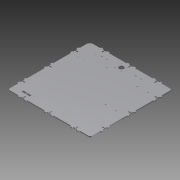
# Autodesk Inventor part: base
Saved by Autodesk Inventor 2012 (Build 160160000, 160)
## iProperties
Created: 2014-12-15
Part Number: base
Material: Default
Document SubType Name: Modeling
Designer: PRINCIPAL
Density: 1 g/cm^3
Author: PRINCIPAL
Autodesk Inventor part; units mm, degrees
ref_plane "YZ Plane" through (0, 0, 0) normal (1, 0, 0) x (0, 1, 0)
ref_plane "XZ Plane" through (0, 0, 0) normal (0, 1, 0) x (-1, 0, 0)
ref_plane "XY Plane" through (0, 0, 0) normal (0, 0, 1) x (1, 0, 0)
sketch "Boceto1" plane through (0, 0, 0) normal (0, 0, 1) x (1, 0, 0)
  arc A0 (118.25, 311.375) -> (118.25, 314.525) centre (118.25, 312.95) ccw
  line L0 (118.25, 311.375) -> (114.65, 311.375)
  arc A1 (114.65, 314.525) -> (114.65, 311.375) centre (114.65, 312.95) ccw
  line L1 (114.65, 314.525) -> (118.25, 314.525)
  arc A2 (93.2214, 311.4) -> (93.2214, 314.5) centre (93.2214, 312.95) ccw
  line L2 (93.2214, 311.4) -> (89.6786, 311.4)
  arc A3 (89.6786, 314.5) -> (89.6786, 311.4) centre (89.6786, 312.95) ccw
  line L3 (89.6786, 314.5) -> (93.2214, 314.5)
  line L4 (251.6786, 314.5) -> (255.2214, 314.5)
  arc A4 (255.2214, 311.4) -> (255.2214, 314.5) centre (255.2214, 312.95) ccw
  line L5 (255.2214, 311.4) -> (251.6786, 311.4)
  arc A5 (251.6786, 314.5) -> (251.6786, 311.4) centre (251.6786, 312.95) ccw
  line L6 (276.6786, 314.5) -> (280.2214, 314.5)
  arc A6 (280.2214, 311.4) -> (280.2214, 314.5) centre (280.2214, 312.95) ccw
  line L7 (280.2214, 311.4) -> (276.6786, 311.4)
  arc A7 (276.6786, 314.5) -> (276.6786, 311.4) centre (276.6786, 312.95) ccw
  arc A8 (184.95, 323.95) -> (173.95, 312.95) centre (184.95, 312.95) ccw
  arc A9 (173.95, 312.95) -> (184.95, 301.95) centre (184.95, 312.95) ccw
  arc A10 (184.95, 301.95) -> (195.95, 312.95) centre (184.95, 312.95) ccw
  arc A11 (195.95, 312.95) -> (184.95, 323.95) centre (184.95, 312.95) ccw
  arc A12 (169.45, 299) -> (167.9, 297.45) centre (169.45, 297.45) ccw
  arc A13 (167.9, 297.45) -> (169.45, 295.9) centre (169.45, 297.45) ccw
  arc A14 (169.45, 295.9) -> (171, 297.45) centre (169.45, 297.45) ccw
  arc A15 (171, 297.45) -> (169.45, 299) centre (169.45, 297.45) ccw
  arc A16 (200.45, 330) -> (198.9, 328.45) centre (200.45, 328.45) ccw
  arc A17 (198.9, 328.45) -> (200.45, 326.9) centre (200.45, 328.45) ccw
  arc A18 (200.45, 326.9) -> (202, 328.45) centre (200.45, 328.45) ccw
  arc A19 (202, 328.45) -> (200.45, 330) centre (200.45, 328.45) ccw
  arc A20 (169.45, 330) -> (167.9, 328.45) centre (169.45, 328.45) ccw
  arc A21 (167.9, 328.45) -> (169.45, 326.9) centre (169.45, 328.45) ccw
  arc A22 (169.45, 326.9) -> (171, 328.45) centre (169.45, 328.45) ccw
  arc A23 (171, 328.45) -> (169.45, 330) centre (169.45, 328.45) ccw
  arc A24 (200.45, 299) -> (198.9, 297.45) centre (200.45, 297.45) ccw
  arc A25 (198.9, 297.45) -> (200.45, 295.9) centre (200.45, 297.45) ccw
  arc A26 (200.45, 295.9) -> (202, 297.45) centre (200.45, 297.45) ccw
  arc A27 (202, 297.45) -> (200.45, 299) centre (200.45, 297.45) ccw
  line L8 (197.9907, 331.1677) -> (197.9907, 334.0126)
  line L9 (197.9907, 334.0126) -> (196.7407, 334.0126)
  line L10 (196.7407, 334.0126) -> (196.7407, 337)
  line L11 (196.7407, 337) -> (197.9907, 337)
  line L12 (197.9907, 337) -> (197.9907, 342.9)
  line L13 (197.9907, 342.9) -> (190.1, 342.9)
  line L14 (190.1, 342.9) -> (190.1, 347.9)
  line L15 (190.1, 347.9) -> (179.8, 347.9)
  line L16 (179.8, 347.9) -> (179.8, 342.9)
  line L17 (179.8, 342.9) -> (95.1, 342.9)
  line L18 (95.1, 342.9) -> (95.1, 347.9)
  line L19 (95.1, 347.9) -> (84.8, 347.9)
  line L20 (84.8, 347.9) -> (84.8, 342.9)
  line L21 (84.8, 342.9) -> (77.1372, 342.9)
  line L22 (77.1372, 342.9) -> (77.1372, 337)
  line L23 (77.1372, 337) -> (78.3872, 337)
  line L24 (78.3872, 337) -> (78.3872, 334.0126)
  line L25 (78.3872, 334.0126) -> (77.1372, 334.0126)
  line L26 (77.1372, 334.0126) -> (77.1372, 329.7126)
  line L27 (77.1372, 329.7126) -> (72.9907, 329.7126)
  line L28 (72.9907, 329.7126) -> (72.9907, 334.0126)
  line L29 (72.9907, 334.0126) -> (71.7407, 334.0126)
  line L30 (71.7407, 334.0126) -> (71.7407, 337)
  line L31 (71.7407, 337) -> (72.9907, 337)
  line L32 (72.9907, 337) -> (72.9907, 342.9)
  line L33 (72.9907, 342.9) -> (65.1, 342.9)
  line L34 (65.1, 342.9) -> (65.1, 347.9)
  line L35 (65.1, 347.9) -> (54.8, 347.9)
  line L36 (54.8, 347.9) -> (54.8, 342.9)
  line L37 (54.8, 342.9) -> (20, 342.9)
  arc A28 (20, 342.9) -> (5, 327.9) centre (20, 327.9) ccw
  line L38 (5, 327.9) -> (5, 294.1)
  line L39 (5, 294.1) -> (0, 294.1)
  line L40 (0, 294.1) -> (0, 283.8)
  line L41 (0, 283.8) -> (5, 283.8)
  line L42 (5, 283.8) -> (5, 275.9744)
  line L43 (5, 275.9744) -> (11.0499, 275.9744)
  line L44 (11.0499, 275.9744) -> (11.0499, 277.2244)
  line L45 (11.0499, 277.2244) -> (14.0508, 277.2244)
  line L46 (14.0508, 277.2244) -> (14.0508, 275.9744)
  line L47 (14.0508, 275.9744) -> (18.5, 275.9744)
  line L48 (18.5, 275.9744) -> (18.5, 271.8605)
  line L49 (18.5, 271.8605) -> (14.0508, 271.8605)
  line L50 (14.0508, 271.8605) -> (14.0508, 270.6105)
  line L51 (14.0508, 270.6105) -> (11.0499, 270.6105)
  line L52 (11.0499, 270.6105) -> (11.0499, 271.8605)
  line L53 (11.0499, 271.8605) -> (5, 271.8605)
  line L54 (5, 271.8605) -> (5, 264.1)
  line L55 (5, 264.1) -> (0, 264.1)
  line L56 (0, 264.1) -> (0, 253.8)
  line L57 (0, 253.8) -> (5, 253.8)
  line L58 (5, 253.8) -> (5, 169.1)
  line L59 (5, 169.1) -> (0, 169.1)
  line L60 (0, 169.1) -> (0, 158.8)
  line L61 (0, 158.8) -> (5, 158.8)
  line L62 (5, 158.8) -> (5, 150.9744)
  line L63 (5, 150.9744) -> (11.0501, 150.9744)
  line L64 (11.0501, 150.9744) -> (11.0501, 152.2244)
  line L65 (11.0501, 152.2244) -> (14.0502, 152.2244)
  line L66 (14.0502, 152.2244) -> (14.0502, 150.9744)
  line L67 (14.0502, 150.9744) -> (18.5, 150.9744)
  line L68 (18.5, 150.9744) -> (18.5, 146.8605)
  line L69 (18.5, 146.8605) -> (14.0502, 146.8605)
  line L70 (14.0502, 146.8605) -> (14.0502, 145.6105)
  line L71 (14.0502, 145.6105) -> (11.0501, 145.6105)
  line L72 (11.0501, 145.6105) -> (11.0501, 146.8605)
  line L73 (11.0501, 146.8605) -> (5, 146.8605)
  line L74 (5, 146.8605) -> (5, 139.1)
  line L75 (5, 139.1) -> (0, 139.1)
  line L76 (0, 139.1) -> (0, 128.8)
  line L77 (0, 128.8) -> (5, 128.8)
  line L78 (5, 128.8) -> (5, 44.074)
  line L79 (5, 44.074) -> (0, 44.074)
  line L80 (0, 44.074) -> (0, 33.774)
  line L81 (0, 33.774) -> (5, 33.774)
  line L82 (5, 33.774) -> (5, 25.9484)
  line L83 (5, 25.9484) -> (11.0521, 25.9484)
  line L84 (11.0521, 25.9484) -> (11.0521, 27.1984)
  line L85 (11.0521, 27.1984) -> (14.0499, 27.1984)
  line L86 (14.0499, 27.1984) -> (14.0499, 25.9484)
  line L87 (14.0499, 25.9484) -> (18.3499, 25.9484)
  line L88 (18.3499, 25.9484) -> (18.3499, 21.8345)
  line L89 (18.3499, 21.8345) -> (14.0499, 21.8345)
  line L90 (14.0499, 21.8345) -> (14.0499, 20.5845)
  line L91 (14.0499, 20.5845) -> (11.0521, 20.5845)
  line L92 (11.0521, 20.5845) -> (11.0521, 21.8345)
  line L93 (11.0521, 21.8345) -> (5, 21.8345)
  line L94 (5, 21.8345) -> (5, 14.074)
  line L95 (5, 14.074) -> (0, 14.074)
  line L96 (0, 14.074) -> (0, 3.774)
  line L97 (0, 3.774) -> (5, 3.774)
  line L98 (5, 3.774) -> (5, -37.026)
  arc A29 (5, -37.026) -> (13, -45.026) centre (13, -37.026) ccw
  line L99 (13, -45.026) -> (54.8, -45.026)
  line L100 (54.8, -45.026) -> (54.8, -50.026)
  line L101 (54.8, -50.026) -> (65.1, -50.026)
  line L102 (65.1, -50.026) -> (65.1, -45.026)
  line L103 (65.1, -45.026) -> (72.9907, -45.026)
  line L104 (72.9907, -45.026) -> (72.9907, -39.126)
  line L105 (72.9907, -39.126) -> (71.7407, -39.126)
  line L106 (71.7407, -39.126) -> (71.7407, -36.1386)
  line L107 (71.7407, -36.1386) -> (72.9907, -36.1386)
  line L108 (72.9907, -36.1386) -> (72.9907, -31.8386)
  line L109 (72.9907, -31.8386) -> (77.1372, -31.8386)
  line L110 (77.1372, -31.8386) -> (77.1372, -36.1386)
  line L111 (77.1372, -36.1386) -> (78.3872, -36.1386)
  line L112 (78.3872, -36.1386) -> (78.3872, -39.126)
  line L113 (78.3872, -39.126) -> (77.1372, -39.126)
  line L114 (77.1372, -39.126) -> (77.1372, -45.026)
  line L115 (77.1372, -45.026) -> (84.8, -45.026)
  line L116 (84.8, -45.026) -> (84.8, -50.026)
  line L117 (84.8, -50.026) -> (95.1, -50.026)
  line L118 (95.1, -50.026) -> (95.1, -45.026)
  line L119 (95.1, -45.026) -> (179.8, -45.026)
  line L120 (179.8, -45.026) -> (179.8, -50.026)
  line L121 (179.8, -50.026) -> (190.1, -50.026)
  line L122 (190.1, -50.026) -> (190.1, -45.026)
  line L123 (190.1, -45.026) -> (197.9907, -45.026)
  line L124 (197.9907, -45.026) -> (197.9907, -39.126)
  line L125 (197.9907, -39.126) -> (196.7407, -39.126)
  line L126 (196.7407, -39.126) -> (196.7407, -36.1386)
  line L127 (196.7407, -36.1386) -> (197.9907, -36.1386)
  line L128 (197.9907, -36.1386) -> (197.9907, -31.8386)
  line L129 (197.9907, -31.8386) -> (202.1372, -31.8386)
  line L130 (202.1372, -31.8386) -> (202.1372, -36.1386)
  line L131 (202.1372, -36.1386) -> (203.3872, -36.1386)
  line L132 (203.3872, -36.1386) -> (203.3872, -39.126)
  line L133 (203.3872, -39.126) -> (202.1372, -39.126)
  line L134 (202.1372, -39.126) -> (202.1372, -45.026)
  line L135 (202.1372, -45.026) -> (209.8, -45.026)
  line L136 (209.8, -45.026) -> (209.8, -50.026)
  line L137 (209.8, -50.026) -> (220.1, -50.026)
  line L138 (220.1, -50.026) -> (220.1, -45.026)
  line L139 (220.1, -45.026) -> (304.8, -45.026)
  line L140 (304.8, -45.026) -> (304.8, -50.026)
  line L141 (304.8, -50.026) -> (315.1, -50.026)
  line L142 (315.1, -50.026) -> (315.1, -45.026)
  line L143 (315.1, -45.026) -> (322.9907, -45.026)
  line L144 (322.9907, -45.026) -> (322.9907, -39.126)
  line L145 (322.9907, -39.126) -> (321.7407, -39.126)
  line L146 (321.7407, -39.126) -> (321.7407, -36.1386)
  line L147 (321.7407, -36.1386) -> (322.9907, -36.1386)
  line L148 (322.9907, -36.1386) -> (322.9907, -31.8386)
  line L149 (322.9907, -31.8386) -> (327.1372, -31.8386)
  line L150 (327.1372, -31.8386) -> (327.1372, -36.1386)
  line L151 (327.1372, -36.1386) -> (328.3872, -36.1386)
  line L152 (328.3872, -36.1386) -> (328.3872, -39.126)
  line L153 (328.3872, -39.126) -> (327.1372, -39.126)
  line L154 (327.1372, -39.126) -> (327.1372, -45.026)
  line L155 (327.1372, -45.026) -> (334.8, -45.026)
  line L156 (334.8, -45.026) -> (334.8, -50.026)
  line L157 (334.8, -50.026) -> (345.1, -50.026)
  line L158 (345.1, -50.026) -> (345.1, -45.026)
  line L159 (345.1, -45.026) -> (386.9, -45.026)
  arc A30 (386.9, -45.026) -> (394.9, -37.026) centre (386.9, -37.026) ccw
  line L160 (394.9, -37.026) -> (394.9, 3.774)
  line L161 (394.9, 3.774) -> (399.9, 3.774)
  line L162 (399.9, 3.774) -> (399.9, 14.074)
  line L163 (399.9, 14.074) -> (394.9, 14.074)
  line L164 (394.9, 14.074) -> (394.9, 21.8345)
  line L165 (394.9, 21.8345) -> (389, 21.8345)
  line L166 (389, 21.8345) -> (389, 20.5845)
  line L167 (389, 20.5845) -> (385.9997, 20.5845)
  line L168 (385.9997, 20.5845) -> (385.9997, 21.8345)
  line L169 (385.9997, 21.8345) -> (381.6997, 21.8345)
  line L170 (381.6997, 21.8345) -> (381.6997, 25.9484)
  line L171 (381.6997, 25.9484) -> (385.9997, 25.9484)
  line L172 (385.9997, 25.9484) -> (385.9997, 27.1984)
  line L173 (385.9997, 27.1984) -> (389, 27.1984)
  line L174 (389, 27.1984) -> (389, 25.9484)
  line L175 (389, 25.9484) -> (394.9, 25.9484)
  line L176 (394.9, 25.9484) -> (394.9, 33.774)
  line L177 (394.9, 33.774) -> (399.9, 33.774)
  line L178 (399.9, 33.774) -> (399.9, 44.074)
  line L179 (399.9, 44.074) -> (394.9, 44.074)
  line L180 (394.9, 44.074) -> (394.9, 128.8)
  line L181 (394.9, 128.8) -> (399.9, 128.8)
  line L182 (399.9, 128.8) -> (399.9, 139.1)
  line L183 (399.9, 139.1) -> (394.9, 139.1)
  line L184 (394.9, 139.1) -> (394.9, 146.8605)
  line L185 (394.9, 146.8605) -> (389, 146.8605)
  line L186 (389, 146.8605) -> (389, 145.6105)
  line L187 (389, 145.6105) -> (385.9997, 145.6105)
  line L188 (385.9997, 145.6105) -> (385.9997, 146.8605)
  line L189 (385.9997, 146.8605) -> (381.6997, 146.8605)
  line L190 (381.6997, 146.8605) -> (381.6997, 150.9744)
  line L191 (381.6997, 150.9744) -> (385.9997, 150.9744)
  line L192 (385.9997, 150.9744) -> (385.9997, 152.2244)
  line L193 (385.9997, 152.2244) -> (389, 152.2244)
  line L194 (389, 152.2244) -> (389, 150.9744)
  line L195 (389, 150.9744) -> (394.9, 150.9744)
  line L196 (394.9, 150.9744) -> (394.9, 158.8)
  line L197 (394.9, 158.8) -> (399.9, 158.8)
  line L198 (399.9, 158.8) -> (399.9, 169.1)
  line L199 (399.9, 169.1) -> (394.9, 169.1)
  line L200 (394.9, 169.1) -> (394.9, 253.8)
  line L201 (394.9, 253.8) -> (399.9, 253.8)
  line L202 (399.9, 253.8) -> (399.9, 264.1)
  line L203 (399.9, 264.1) -> (394.9, 264.1)
  line L204 (394.9, 264.1) -> (394.9, 271.8605)
  line L205 (394.9, 271.8605) -> (389, 271.8605)
  line L206 (389, 271.8605) -> (389, 270.6105)
  line L207 (389, 270.6105) -> (385.9997, 270.6105)
  line L208 (385.9997, 270.6105) -> (385.9997, 271.8605)
  line L209 (385.9997, 271.8605) -> (381.6997, 271.8605)
  line L210 (381.6997, 271.8605) -> (381.6997, 275.9744)
  line L211 (381.6997, 275.9744) -> (385.9997, 275.9744)
  line L212 (385.9997, 275.9744) -> (385.9997, 277.2244)
  line L213 (385.9997, 277.2244) -> (389, 277.2244)
  line L214 (389, 277.2244) -> (389, 275.9744)
  line L215 (389, 275.9744) -> (394.9, 275.9744)
  line L216 (394.9, 275.9744) -> (394.9, 283.8)
  line L217 (394.9, 283.8) -> (399.9, 283.8)
  line L218 (399.9, 283.8) -> (399.9, 294.1)
  line L219 (399.9, 294.1) -> (394.9, 294.1)
  line L220 (394.9, 294.1) -> (394.9, 332.9)
  arc A31 (394.9, 332.9) -> (384.9, 342.9) centre (384.9, 332.9) ccw
  line L221 (384.9, 342.9) -> (345.1, 342.9)
  line L222 (345.1, 342.9) -> (345.1, 347.9)
  line L223 (345.1, 347.9) -> (334.8, 347.9)
  line L224 (334.8, 347.9) -> (334.8, 342.9)
  line L225 (334.8, 342.9) -> (327.1372, 342.9)
  line L226 (327.1372, 342.9) -> (327.1372, 337)
  line L227 (327.1372, 337) -> (328.3872, 337)
  line L228 (328.3872, 337) -> (328.3872, 334.0126)
  line L229 (328.3872, 334.0126) -> (327.1372, 334.0126)
  line L230 (327.1372, 334.0126) -> (327.1372, 329.7126)
  line L231 (327.1372, 329.7126) -> (322.9907, 329.7126)
  line L232 (322.9907, 329.7126) -> (322.9907, 334.0126)
  line L233 (322.9907, 334.0126) -> (321.7407, 334.0126)
  line L234 (321.7407, 334.0126) -> (321.7407, 337)
  line L235 (321.7407, 337) -> (322.9907, 337)
  line L236 (322.9907, 337) -> (322.9907, 342.9)
  line L237 (322.9907, 342.9) -> (315.1, 342.9)
  line L238 (315.1, 342.9) -> (315.1, 347.9)
  line L239 (315.1, 347.9) -> (304.8, 347.9)
  line L240 (304.8, 347.9) -> (304.8, 342.9)
  line L241 (304.8, 342.9) -> (220.1, 342.9)
  line L242 (220.1, 342.9) -> (220.1, 347.9)
  line L243 (220.1, 347.9) -> (209.8, 347.9)
  line L244 (209.8, 347.9) -> (209.8, 342.9)
  line L245 (209.8, 342.9) -> (202.1372, 342.9)
  line L246 (202.1372, 342.9) -> (202.1372, 337)
  line L247 (202.1372, 337) -> (203.3872, 337)
  line L248 (203.3872, 337) -> (203.3872, 334.0126)
  line L249 (203.3872, 334.0126) -> (202.1372, 334.0126)
  line L250 (202.1372, 334.0126) -> (202.1372, 331.1677)
  line L251 (202.1372, 331.1677) -> (197.9907, 331.1677)
  arc A32 (35.6101, 256.5465) -> (34.0601, 254.9965) centre (35.6101, 254.9965) ccw
  arc A33 (34.0601, 254.9965) -> (35.6101, 253.4465) centre (35.6101, 254.9965) ccw
  arc A34 (35.6101, 253.4465) -> (37.1601, 254.9965) centre (35.6101, 254.9965) ccw
  arc A35 (37.1601, 254.9965) -> (35.6101, 256.5465) centre (35.6101, 254.9965) ccw
  arc A36 (63.7111, 256.5465) -> (62.1611, 254.9965) centre (63.7111, 254.9965) ccw
  arc A37 (62.1611, 254.9965) -> (63.7111, 253.4465) centre (63.7111, 254.9965) ccw
  arc A38 (63.7111, 253.4465) -> (65.2611, 254.9965) centre (63.7111, 254.9965) ccw
  arc A39 (65.2611, 254.9965) -> (63.7111, 256.5465) centre (63.7111, 254.9965) ccw
  arc A40 (68.6905, 309.0473) -> (66.9405, 307.2973) centre (68.6905, 307.2973) ccw
  arc A41 (66.9405, 307.2973) -> (68.6905, 305.5473) centre (68.6905, 307.2973) ccw
  arc A42 (68.6905, 305.5473) -> (70.4405, 307.2973) centre (68.6905, 307.2973) ccw
  arc A43 (70.4405, 307.2973) -> (68.6905, 309.0473) centre (68.6905, 307.2973) ccw
  line L252 (45.3508, -23.0317) -> (64.3508, -23.0317)
  line L253 (64.3508, -23.0317) -> (64.3508, -14.0317)
  line L254 (64.3508, -14.0317) -> (45.3508, -14.0317)
  line L255 (45.3508, -14.0317) -> (45.3508, -23.0317)
  line L256 (67.0064, -23.0635) -> (86.0064, -23.0635)
  line L257 (86.0064, -23.0635) -> (86.0064, -14.0635)
  line L258 (86.0064, -14.0635) -> (67.0064, -14.0635)
  line L259 (67.0064, -14.0635) -> (67.0064, -23.0635)
  point P0 (0, 0)
  point P1 (184.95, 312.95)
  dimension "d10" = 21.4286
  dimension "d11" = 21.4571
  dimension "d12" = 3.5429
  dimension "d13" = 3.5429
  dimension "d14" = 3.5429
  dimension "d15" = 3.6
  dimension "d22" = 0
  dimension "d23" = 0
  constraints: 520 end point, 88 point on circle, 44 centre point
  measures "d10" distance of A2.centre A1.centre
  measures "d11" distance of A7.centre A4.centre
  measures "d12" distance of A7.centre A6.centre
  measures "d13" distance of A4.centre A5.centre
  measures "d14" distance of A2.centre A3.centre
  measures "d15" distance of A0.centre A1.centre
  measures "d22" distance of point (280.221, 312.95) A6.centre
  measures "d23" distance of point (89.679, 312.95) A3.centre
extrude "Extrusión1" add sketch "Boceto1" along normal blind 5
sketch "Boceto2" plane through (0, 0, 5) normal (0, 0, 1) x (1, 0, 0)
  line L0 (95.1, 342.9) -> (179.8, 342.9) projected
  line L1 (5, 44.074) -> (5, 128.8) projected
  circle A0 centre (150.75, 278.15) radius 1.75
  point P0 (0, 0)
  dimension "d2" = 3.5
  dimension "d3" = 145.75
  dimension "d5" = 64.75
  constraints: 1 centre point
  measures "d2" diameter of A0
  measures "d3" distance from line of A0.centre L1
  measures "d5" distance from line of A0.centre L0
extrude "Extrusión2" cut sketch "Boceto2" against normal blind 10
sketch "Boceto3" plane through (0, 0, 5) normal (0, 0, 1) x (1, 0, 0)
  line L0 (220.1, 342.9) -> (304.8, 342.9) projected
  circle A0 centre (299.9, 272.9) radius 2.275
  circle A1 centre (299.9, 122.9) radius 2.25
  circle A2 centre (349.9, 122.9) radius 2.25
  circle A3 centre (349.9, 272.9) radius 2.25
  point P0 (399.9, 264.1)
  point P1 (0, 0)
  dimension "d24" = 4.55
  dimension "d25" = 4.5
  dimension "d26" = 4.5
  dimension "d27" = 4.5
  dimension "d28" = 150
  dimension "d29" = 150
  dimension "d30" = 50
  dimension "d31" = 70
  dimension "d32" = 50
  constraints: 4 centre point
  measures "d24" diameter of A0
  measures "d25" diameter of A1
  measures "d26" diameter of A2
  measures "d27" diameter of A3
  measures "d28" distance of A1.centre A0.centre
  measures "d29" distance of A2.centre A3.centre
  measures "d30" distance of A2.centre A1.centre
  measures "d31" distance from line of L0 A3.centre
  measures "d32" horizontal distance of point (399.9, 264.1) A3.centre
extrude "Extrusión3" cut sketch "Boceto3" against normal blind 10
